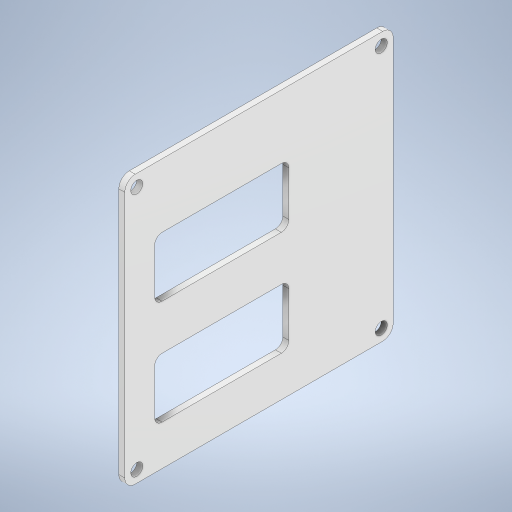
# Autodesk Inventor part: RightCover
Saved by Autodesk Inventor 2024 (Build 280153000, 153)
## iProperties
Created: 2023-11-23
Part Number: RightCover
Material: ABS Plastic
Document SubType Name: Modeling
Designer: G2O
Density: 1.06 g/cm^3
Appearance: Smooth - White
Author: G2O
Autodesk Inventor part; units mm, degrees
ref_plane "YZ Plane" through (0, 0, 0) normal (1, 0, 0) x (0, 1, 0)
ref_plane "XZ Plane" through (0, 0, 0) normal (0, 1, 0) x (-1, 0, 0)
ref_plane "XY Plane" through (0, 0, 0) normal (0, 0, 1) x (1, 0, 0)
sketch "Sketch1" plane through (0, 0, 0) normal (1, 0, 0) x (0, 1, 0)
  line L0 (45, 45) -> (-45, 45)
  line L1 (-45, 45) -> (-45, -45)
  line L2 (-45, -45) -> (45, -45)
  line L3 (45, -45) -> (45, 45)
  line L4 (45, 45) -> (-45, -45) construction
  line L5 (-45, 45) -> (45, -45) construction
  point P0 (0, 0)
  dimension "d0" = 90
  dimension "d1" = 90
  constraints: 12 end point, 2 midpoint, 2 parallel, 1 horizontal, 1 perpendicular
  measures "d0" distance of L2.end L1.end
  measures "d1" distance of L1.end L0.end
extrude "Extrusion1" add sketch "Sketch1" along normal blind 2
sketch "Sketch2" plane through (2, 0, 0) normal (1, 0, 0) x (0, 0, -1)
  line L0 (45, 45) -> (-45, 45) projected
  line L1 (-45, 45) -> (-41, 45)
  line L2 (-41, 45) -> (-41, 41)
  circle A0 centre (-41, 41) radius 2
  line L3 (45, -45) -> (45, 45) projected
  line L4 (45, 45) -> (41, 45)
  line L5 (41, 45) -> (41, 41)
  circle A1 centre (41, 41) radius 2
  line L6 (-45, 45) -> (-45, -45) projected
  line L7 (-45, -45) -> (-41, -45)
  line L8 (-45, -45) -> (45, -45) projected
  line L9 (-41, -45) -> (-41, -41)
  circle A2 centre (-41, -41) radius 2
  line L10 (45, -45) -> (41, -45)
  line L11 (41, -45) -> (41, -41)
  circle A3 centre (41, -41) radius 2
  point P0 (0, 0)
  dimension "d4" = 4
  dimension "d5" = 4
  dimension "d6" = 4
  dimension "d7" = 4
  dimension "d8" = 4
  dimension "d9" = 4
  dimension "d10" = 4
  dimension "d11" = 4
  dimension "d12" = 4
  dimension "d13" = 4
  dimension "d14" = 4
  dimension "d15" = 4
  constraints: 16 end point, 4 centre point, 4 coincident, 4 point on line, 2 perpendicular, 2 vertical
  measures "d4" distance of L0.end L1.end
  measures "d5" distance of L1.end L2.end
  measures "d6" diameter of A0
  measures "d7" distance of L0.start L4.end
  measures "d8" distance of L4.end L5.end
  measures "d9" diameter of A1
  measures "d10" distance of L6.end L7.end
  measures "d11" distance of L7.end L9.end
  measures "d12" diameter of A2
  measures "d13" distance of L3.start L10.end
  measures "d14" distance of L10.end L11.end
  measures "d15" diameter of A3
extrude "Extrusion2" cut sketch "Sketch2" against normal up to surface (2 mm away) contours A1 | A0 | A2 | A3
fillet "Fillet1" radius 3.5 4 edges at (1, 45, -45) (1, -45, -45) (1, -45, 45) (1, 45, 45)
sketch "Sketch3" plane through (2, 0, 0) normal (1, 0, 0) x (0, 0, -1)
  line L0 (-41.5, -45) -> (41.5, -45) projected
  line L1 (0, -45) -> (0, -41.5)
  line L2 (0, -41.5) -> (0, -31.5)
  line L3 (0, -31.5) -> (0, -11.5)
  line L4 (0, -45) -> (0, -6.37)
  line L5 (0, -6.37) -> (0, 3.63)
  line L6 (0, 3.63) -> (0, 23.63)
  line L7 (45, -41.5) -> (45, 41.5) projected
  line L8 (45, 0) -> (10, 0)
  line L9 (10, 0) -> (10, 3.63)
  line L10 (10, 3.63) -> (-35, 3.63)
  line L11 (-35, 3.63) -> (-35, 23.63)
  line L12 (-35, 23.63) -> (10, 23.63)
  line L13 (10, 23.63) -> (10, 3.63)
  line L14 (10, 0) -> (10, -11.5)
  line L15 (10, -11.5) -> (-35, -11.5)
  line L16 (-35, -11.5) -> (-35, -31.5)
  line L17 (-35, -31.5) -> (10, -31.5)
  line L18 (10, -31.5) -> (10, -11.5)
  point P0 (0, 0)
  dimension "d19" = 3.5
  dimension "d20" = 10
  dimension "d21" = 20
  dimension "d22" = 38.63
  dimension "d23" = 10
  dimension "d24" = 20
  dimension "d25" = 35
  dimension "d26" = 45
  dimension "d27" = 20
  dimension "d28" = 45
  dimension "d29" = 20
  constraints: 34 end point, 5 vertical, 4 parallel, 3 horizontal, 3 point on line, 2 midpoint, 2 perpendicular
  measures "d19" distance of L1.start L1.end
  measures "d20" distance of L1.end L2.end
  measures "d21" distance of L2.end L3.end
  measures "d22" distance of L1.start L4.end
  measures "d23" distance of L4.end L5.end
  measures "d24" distance of L5.end L6.end
  measures "d25" distance of L8.start L8.end
  measures "d26" distance of L11.end L12.end
  measures "d27" distance of L10.end L11.end
  measures "d28" distance of L17.end L16.end
  measures "d29" distance of L16.end L15.end
extrude "Extrusion3" cut sketch "Sketch3" against normal up to surface (2 mm away) contours L17 L16 L15 L3 | L3 L15 L18 L17 | L10 L11 L12 L6 | L6 L12 L13 L10
fillet "Fillet2" radius 2.5 8 edges at (1, 23.63, -10) (1, -11.5, -10) (1, 23.63, 35) (1, -11.5, 35) (1, 3.63, -10) (1, -31.5, -10) (1, 3.63, 35) (1, -31.5, 35)
body "Solid1"
